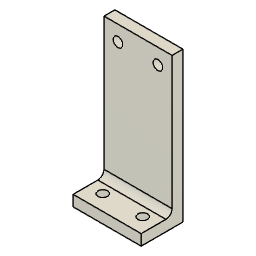
Alcohol+valve+mount (Autodesk Fusion 360 archive; units mm, degrees)
design "Alcohol valve mount"
Autodesk Fusion 360 part; units mm, degrees
sketch "Sketch1" plane through (0, 0, 0) normal (0, 1, 0) x (1, 0, 0)
  line L0 (0, 0) -> (22, 0)
  line L1 (22, 0) -> (22, -13.5)
  line L2 (22, -13.5) -> (0, -13.5)
  line L3 (0, -13.5) -> (0, 0)
  line L4 (0, -3.5) -> (22, -3.5)
  line L5 (0, -8.5) -> (22, -8.5) construction
  circle A0 centre (4.6, -8.5) radius 1.55
  circle A1 centre (17.5, -8.5) radius 1.55
  dimension "d1" = 22
  dimension "d2" = 13.5
  dimension "d3" = 3.5
  dimension "d4" = 5
  dimension "d5" = 3.1
  dimension "d6" = 3.1
  dimension "d7" = 12.9
  dimension "d8" = 4.5
  constraint horizontal L0
  constraint vertical L1
  constraint horizontal L2
  constraint vertical L3
  constraint coincident L0.start L3.end
  constraint coincident L3 L4.start
  constraint coincident L1 L4.end
  constraint perpendicular L1 L4
  constraint coincident L3 L5.start
  constraint coincident L1 L5.end
  constraint perpendicular L1 L5
  constraint coincident L5 A0.centre
  constraint coincident L5 A1.centre
  measures "d1" distance of L0.start L0.end
  measures "d2" distance of L0.start L2.end
  measures "d3" distance of L0 L4
  measures "d4" distance of L2 L5
  measures "d5" diameter of A0
  measures "d6" diameter of A1
  measures "d7" distance of A0.centre A1.centre
  measures "d8" distance of L1 A1.centre
extrude "Extrude1" add sketch "Sketch1" along normal blind 3.5 contours L1 L2 L3 L4
extrude "Extrude2" add sketch "Sketch1" along normal blind 48.4 contours L0 L1 L3 L4
sketch "Sketch2" plane through (0, 0, 0) normal (0, 0, -1) x (-1, 0, 0)
  line L0 (-22, 0) -> (0, 0)
  line L1 (0, 0) -> (0, 48.4)
  line L2 (0, 48.4) -> (-22, 48.4)
  line L3 (-22, 48.4) -> (-22, 0)
  line L4 (-22, 43.4) -> (0, 43.4) construction
  line L5 (0, 0) -> (-22, 0)
  circle A0 centre (-17.4, 43.4) radius 1.55
  circle A1 centre (-4.5, 43.4) radius 1.55
  dimension "d13" = 43.4
  dimension "d14" = 3.1
  dimension "d15" = 3.1
  dimension "d16" = 12.9
  dimension "d17" = 4.5
  constraint coincident L3 L4.start
  constraint coincident L1 L4.end
  constraint perpendicular L1 L4
  constraint coincident L4 A0.centre
  constraint coincident L4 A1.centre
  measures "d13" distance of L4 L5
  measures "d14" diameter of A0
  measures "d15" diameter of A1
  measures "d16" distance of A0.centre A1.centre
  measures "d17" distance of L1 A1.centre
extrude "Extrude3" cut sketch "Sketch2" against normal up to surface (3.5 mm away) contours A0 | A1
fillet "Fillet1" radius 2 1 edges at (11, 3.5, 3.5)
